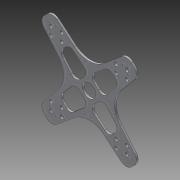
# Autodesk Inventor part: 6061 Bed
Saved by Autodesk Inventor 2014 (Build 180170000, 170)
## iProperties
Created: 2016-05-10
Part Number: 6061 Bed
Material: Aluminum 6061
Document SubType Name: Modeling
Designer: 101767
Density: 2.71 g/cm^3
Appearance: Aluminum - Flat
Mass: 1521.5 g
Surface Area: 1910.74 cm^2
Volume: 561.441 cm^3
Author: 101767
Autodesk Inventor part; units mm, degrees
ref_plane "YZ Plane" through (0, 0, 0) normal (1, 0, 0) x (0, 1, 0)
ref_plane "XZ Plane" through (0, 0, 0) normal (0, 1, 0) x (-1, 0, 0)
ref_plane "XY Plane" through (0, 0, 0) normal (0, 0, 1) x (1, 0, 0)
sketch "Plate" plane through (0, 0, 0) normal (0, 0, 1) x (1, 0, 0)
  line L0 (-100, -100) -> (100, -100) construction
  line L1 (100, -100) -> (100, 100) construction
  line L2 (100, 100) -> (-100, 100) construction
  line L3 (-100, 100) -> (-100, -100) construction
  line L4 (-100, -100) -> (100, 100) construction
  line L5 (100, -100) -> (-100, 100) construction
  line L6 (0, 0) -> (0, 420.657) construction
  line L7 (0, 0) -> (461.6465, 0) construction
  line L8 (0, 102) -> (102, 102) construction
  line L9 (102, 102) -> (102, 0) construction
  line L10 (48.2756, 0) -> (155.194, 127.4203) construction
  line L11 (154.8388, 45.1612) -> (58.001, 141.999) construction
  line L12 (152.9755, 75.3088) -> (79.3809, 148.9034) construction
  line L13 (48.2756, 0) -> (130.4056, 97.8787)
  line L14 (100, 100) -> (231.4665, 231.4665) construction
  line L15 (130.4056, 97.8787) -> (114.1421, 114.1421)
  line L16 (97.8787, 130.4056) -> (114.1421, 114.1421)
  line L17 (97.8787, 130.4056) -> (0, 48.2756)
  line L18 (-48.2756, 0) -> (-130.4056, 97.8787)
  line L19 (-130.4056, 97.8787) -> (-114.1421, 114.1421)
  line L20 (-97.8787, 130.4056) -> (-114.1421, 114.1421)
  line L21 (-97.8787, 130.4056) -> (0, 48.2756)
  line L22 (48.2756, 0) -> (130.4056, -97.8787)
  line L23 (130.4056, -97.8787) -> (114.1421, -114.1421)
  line L24 (97.8787, -130.4056) -> (114.1421, -114.1421)
  line L25 (97.8787, -130.4056) -> (0, -48.2756)
  line L26 (-97.8787, -130.4056) -> (0, -48.2756)
  line L27 (-97.8787, -130.4056) -> (-114.1421, -114.1421)
  line L28 (-130.4056, -97.8787) -> (-114.1421, -114.1421)
  line L29 (-48.2756, 0) -> (-130.4056, -97.8787)
  dimension "d167" = 3.3
  dimension "d12" = 100
  dimension "d79" = 100
  dimension "d80" = 2
  dimension "d81" = 2
  dimension "d83" = 20
  dimension "d84" = 5
  dimension "d85" = 23
  dimension "d86" = 5
  constraints: 60 end point, 12 symmetric about line, 9 point on line, 5 parallel, 5 perpendicular, 2 midpoint, 1 horizontal
  measures "d12" distance between parallel lines of L7 L2
  measures "d79" distance from line of L1.end L6
  measures "d80" distance between parallel lines of L2 L8
  measures "d81" distance between parallel lines of L1 L9
  measures "d83" distance between parallel lines of L11 L12
  measures "d84" angle of L10 L4
  measures "d85" distance from line of L14 L13.end
  measures "d86" angle of L4 L17
extrude "Base" add sketch "Plate" along normal blind 4.7625
sketch "Sketch3" plane through (0, 0, 0) normal (0, 0, 1) x (1, 0, 0)
  line L0 (0, 48.2756) -> (0, -62.1517) construction
  line L1 (48.2756, 0) -> (-54.0345, 0) construction
  circle A0 centre (0, 0) radius 17.5
  dimension "d150" = 35
  constraints: 4 end point, 2 point on line, 1 centre point, 1 perpendicular, 1 vertical
  measures "d150" diameter of A0
extrude "Center hole" cut sketch "Sketch3" along normal through all
fillet "Fillet2" radius 60 4 edges at (0, 48.2756, 2.3813) (-48.2756, 0, 2.3813) (0, -48.2756, 2.3813) (48.2756, 0, 2.3813)
fillet "Fillet4" radius 20 8 edges at (97.8787, 130.4056, 2.3813) (130.4056, 97.8787, 2.3813) (130.4056, -97.8787, 2.3813) (97.8787, -130.4056, 2.3813) (-97.8787, -130.4056, 2.3813) (-130.4056, -97.8787, 2.3813) (-97.8787, 130.4056, 2.3813) (-130.4056, 97.8787, 2.3813)
sketch "Sketch14" plane through (0, 0, 0) normal (0, 0, 1) x (1, 0, 0)
  line L0 (0, 0) -> (-162.672, 0) construction
  point P0 (-7, 60)
  point P1 (-7, -60)
  dimension "d117" = 7
  dimension "d118" = 60
  constraints: 2 end point, 1 horizontal, 1 symmetric about line
  measures "d117" horizontal distance of L0.start point (-7, 60)
  measures "d118" vertical distance of L0.start point (-7, 60)
hole "Hole5" at (-7, 60, 0) at (-7, -60, 0) direction (0, 0, 1) diameter 4.2 end through all
sketch "Sketch17" plane through (0, 0, 0) normal (0, 0, 1) x (1, 0, 0)
  line L0 (-100, -100) -> (100, 100) construction
  line L1 (154.8388, 45.1612) -> (58.001, 141.999) construction
  line L2 (64.6447, 64.6447) -> (51.1488, 78.1405)
  line L3 (51.1488, 78.1405) -> (1.1657, 36.1997)
  line L4 (1.1657, 36.1997) -> (18.6827, 18.6827)
  line L5 (83.8397, 118.6255) -> (38.5673, 80.6374) construction
  line L6 (64.6447, 64.6447) -> (78.1405, 51.1488)
  line L7 (78.1405, 51.1488) -> (36.1997, 1.1657)
  line L8 (36.1997, 1.1657) -> (18.6827, 18.6827)
  point P0 (0, 0)
  point P1 (38.5673, 80.6374)
  point P2 (0.4229, 70.2877)
  dimension "d133" = 10
  dimension "d134" = 50
  dimension "d135" = 65
  constraints: 12 end point, 2 point on line, 2 symmetric about line, 1 parallel, 1 perpendicular, 2 other
  measures "d134" distance between parallel lines of L2 L1
  measures "d135" distance between parallel lines of L2 L4
extrude "Extrusion4" cut sketch "Sketch17" along normal through all
fillet "Fillet5" radius 15 4 edges at (51.1488, 78.1405, 2.3813) (78.1405, 51.1488, 2.3813) (36.1997, 1.1657, 2.3813) (1.1657, 36.1997, 2.3813)
pattern_circular "Circular Pattern2" count 4 over 360 about axis through (0, 0, -10) along (0, 0, 1) of "Extrusion4", "Fillet5"
sketch "Sketch19" plane through (0, 0, 0) normal (0, 0, 1) x (1, 0, 0)
  line L0 (159.3873, 85) -> (27.6283, 85) construction
  line L1 (85, 174.6938) -> (85, 19.7093) construction
  circle A0 centre (71, 95.5) radius 2.75
  circle A1 centre (99, 95.5) radius 2.75
  circle A2 centre (71, 74.5) radius 2.75
  circle A3 centre (99, 74.5) radius 2.75
  point P0 (0, 0)
  dimension "d151" = 85
  dimension "d152" = 85
  dimension "d153" = 5.5
  dimension "d154" = 14
  dimension "d155" = 10.5
  constraints: 4 centre point, 4 end point, 3 symmetric about line, 1 horizontal, 1 perpendicular, 3 other
  measures "d151" distance from line of L0 point (0, 0)
  measures "d152" distance from line of point (0, 0) L1
  measures "d153" diameter of A0
  measures "d154" distance from line of L1 A0.centre
  measures "d155" distance from line of L0 A0.centre
extrude "Extrusion6" cut sketch "Sketch19" along normal through all
chamfer "Chamfer2" distance 2 angle 45 4 edges at (68.25, 74.5, 4.7625) (96.25, 74.5, 4.7625) (96.25, 95.5, 4.7625) (68.25, 95.5, 4.7625)
pattern_linear "Rectangular Pattern2" count 2 spacing 170 along (-1, 0, 0) count 2 spacing 170 along (0, -1, 0) of "Extrusion6", "Chamfer2"
sketch "Sketch20" plane through (0, 0, 0) normal (0, 0, 1) x (1, 0, 0)
  circle A0 centre (-87, 102) radius 1.65 construction
  arc A1 (-99.8, 102) -> (-102, 99.8) centre (-102, 102) ccw construction
  circle A2 centre (-102, 87) radius 1.65 construction
  circle A3 centre (-87, 102) radius 1.25
  circle A4 centre (-102, 87) radius 1.25
  circle A5 centre (-102, 102) radius 1.65
  point P0 (0, 0)
  dimension "d167" = 3.3
  dimension "d168" = 2.5
  dimension "d169" = 2.5
  constraints: 3 centre point, 3 coincident
  measures "d167" diameter of A5
  measures "d168" diameter of A3
  measures "d169" diameter of A4
extrude "Extrusion7" cut sketch "Sketch20" along normal through all
pattern_circular "Circular Pattern3" count 4 over 360 about axis through (0, 0, -10) along (0, 0, 1) of "Extrusion7"
body "Solid1"
